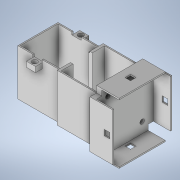
# Autodesk Inventor part: shell 2.0
Saved by Autodesk Inventor 2020.2 (Build 242310000, 310)
## iProperties
Created: 2020-02-10
Part Number: shell 2.0
Material: Generic
Document SubType Name: Modeling
Designer: ColinP
Density: 1 g/cm^3
Appearance: Default
Author: ColinP
Autodesk Inventor part; units mm, degrees
ref_plane "YZ Plane" through (0, 0, 0) normal (1, 0, 0) x (0, 1, 0)
ref_plane "XZ Plane" through (0, 0, 0) normal (0, 1, 0) x (-1, 0, 0)
ref_plane "XY Plane" through (0, 0, 0) normal (0, 0, 1) x (1, 0, 0)
sketch "Sketch1" plane through (0, 0, 0) normal (0, 1, 0) x (-1, 0, 0)
  line L0 (9.0944, 11.3049) -> (-22.9063, 11.3049)
  line L1 (9.0944, 11.3049) -> (41.0951, 11.3049) construction
  line L2 (-22.9063, 11.3049) -> (-22.9063, -19.1751)
  line L3 (-22.9063, -19.1751) -> (9.0944, -19.1751)
  line L4 (9.0944, -19.1751) -> (9.0944, 11.3049)
  point P0 (0, 0)
  dimension "d0" = 32.0007
  dimension "d1" = 180
  dimension "d2" = 30.48
  constraints: 10 end point, 2 horizontal, 2 perpendicular, 1 collinear, 1 vertical
  measures "d0" distance of L0.start L0.end
  measures "d1" angle of L0 L1
  measures "d2" distance of L0.end L2.end
extrude "Extrusion1" add sketch "Sketch1" along normal blind 2
sketch "Sketch2" plane through (0, 2, 0) normal (0, 1, 0) x (1, 0, 0)
  line L0 (-9.0944, 19.1751) -> (-9.0944, -11.3049) projected
  line L1 (-9.0944, -11.3049) -> (-9.0944, -10.3049)
  line L2 (-9.0944, -10.3049) -> (-8.0944, -10.3049)
  line L3 (-9.0944, 19.1751) -> (-8.0944, 19.1751)
  line L4 (22.9063, 19.1751) -> (-9.0944, 19.1751) projected
  line L5 (-8.0944, 19.1751) -> (-8.0944, 18.1751)
  line L6 (22.9063, 19.1751) -> (21.9063, 19.1751)
  line L7 (21.9063, 19.1751) -> (21.9063, 18.1751)
  line L8 (22.9063, -11.3049) -> (22.9063, 19.1751) projected
  line L9 (22.9063, -11.3049) -> (22.9063, -10.3049)
  line L10 (21.9063, -10.3049) -> (22.9063, -10.3049)
  line L11 (-8.0944, -10.3049) -> (21.9063, -10.3049)
  line L12 (21.9063, -10.3049) -> (21.9063, 18.1751)
  line L13 (21.9063, 18.1751) -> (-8.0944, 18.1751)
  line L14 (-8.0944, 18.1751) -> (-8.0944, -10.3049)
  line L15 (-9.0944, -11.3049) -> (22.9063, -11.3049) projected
  line L16 (22.9063, -11.3049) -> (22.9063, 19.1751) projected
  line L17 (22.9063, 19.1751) -> (-9.0944, 19.1751) projected
  line L18 (-9.0944, 19.1751) -> (-9.0944, -11.3049) projected
  line L19 (22.9063, -11.3049) -> (22.9063, -3.3649)
  line L20 (22.9063, 19.1751) -> (22.9063, 11.2351)
  line L21 (22.9063, -3.3649) -> (21.9063, -3.3649)
  line L22 (22.9063, 11.2351) -> (21.9063, 11.2351)
  point P0 (0, 0)
  point P1 (22.9063, -3.3649)
  point P2 (22.9063, 11.2351)
  dimension "d5" = 1
  dimension "d6" = 1
  dimension "d7" = 1
  dimension "d8" = 1
  dimension "d11" = 7.94
  dimension "d12" = 7.94
  constraints: 32 end point, 8 point on line, 6 perpendicular, 2 parallel, 1 horizontal, 1 vertical
  measures "d5" distance of L0.end L1.end
  measures "d6" distance of L1.end L2.end
  measures "d7" distance of L3.end L5.end
  measures "d8" distance of L4.start L6.end
  measures "d11" distance of L15.end L19.end
  measures "d12" distance of L16.end L20.end
extrude "Extrusion3" add sketch "Sketch2" along normal blind 30 contours L3 L5 L14 L2 L0 | L2 L11 L10 L8 L15 L0 | L4 L7 L13 L5 | L4 L8 L22 L12 L7 | L12 L21 L8 L10
sketch "Sketch3" plane through (0, 2, 0) normal (0, 1, 0) x (1, 0, 0)
  line L0 (21.9063, -10.3049) -> (21.9063, -3.3649) projected
  line L1 (22.9063, 11.2351) -> (21.9063, 11.2351) projected
  line L2 (21.9063, -3.3649) -> (21.9063, 11.2351)
  line L3 (21.9063, 11.2351) -> (22.9063, 11.2351)
  line L4 (22.9063, -3.3649) -> (22.9063, 11.2351) projected
  line L5 (22.9063, 11.2351) -> (22.9063, -3.3649)
  line L6 (22.9063, -3.3649) -> (21.9063, -3.3649)
  point P0 (0, 0)
  constraints: 8 end point, 3 perpendicular, 1 vertical
extrude "Extrusion4" add sketch "Sketch3" along normal blind 2
sketch "Sketch4" plane through (0, 32, 0) normal (0, 1, 0) x (1, 0, 0)
  line L0 (22.9063, -11.3049) -> (22.9063, 19.1751) projected
  line L1 (22.9063, 3.9351) -> (5.9063, 3.9351)
  line L2 (5.9063, 3.9351) -> (5.9063, 21.4351)
  line L3 (5.9063, 21.4351) -> (5.9063, -13.5649)
  circle A0 centre (5.9063, -13.5649) radius 2
  circle A1 centre (5.9063, 21.4351) radius 2
  line L4 (22.9063, 19.1751) -> (-9.0944, 19.1751) projected
  line L5 (5.9063, 19.1751) -> (2.4063, 19.1751)
  line L6 (2.4063, 19.1751) -> (2.4063, 24.1751)
  line L7 (2.4063, 24.1751) -> (9.4063, 24.1751)
  line L8 (9.4063, 24.1751) -> (9.4063, 19.1751)
  line L9 (9.4063, -11.3049) -> (9.4063, -16.3049)
  line L10 (9.4063, -16.3049) -> (2.4063, -16.3049)
  line L11 (2.4063, -16.3049) -> (2.4063, -11.3049)
  line L12 (-9.0944, -11.3049) -> (22.9063, -11.3049) projected
  point P0 (0, 0)
  dimension "d17" = 17
  dimension "d18" = 17.5
  dimension "d19" = 35
  dimension "d20" = 4
  dimension "d21" = 4
  dimension "d22" = 3.5
  dimension "d23" = 5
  dimension "d24" = 7
  dimension "d25" = 5
  constraints: 20 end point, 10 point on line, 5 perpendicular, 2 centre point, 2 coincident, 1 horizontal, 1 midpoint
  measures "d17" distance of L1.start L1.end
  measures "d18" distance of L1.end L2.end
  measures "d19" distance of L2.end L3.end
  measures "d20" diameter of A0
  measures "d21" diameter of A1
  measures "d22" distance of L5.start L5.end
  measures "d23" distance of L5.end L6.end
  measures "d24" distance of L6.end L7.end
  measures "d25" distance of L9.start L9.end
extrude "Extrusion5" add sketch "Sketch4" against normal blind 4 contours L9 L10 L11 L12 | L4 L6 L7 L8
sketch "Sketch5" plane through (0, 32, 0) normal (0, 1, 0) x (1, 0, 0)
  line L0 (2.4063, 19.1751) -> (2.4063, 24.1751) projected
  line L1 (2.4063, 19.1751) -> (2.4063, 18.1751)
  line L2 (-8.0944, 18.1751) -> (21.9063, 18.1751) projected
  line L3 (22.9063, 19.1751) -> (9.4063, 19.1751) projected
  line L4 (9.4063, 19.1751) -> (9.4063, 18.1751)
  line L5 (-9.0944, -11.3049) -> (22.9063, -11.3049) projected
  line L6 (2.4063, -11.3049) -> (2.4063, -10.3049)
  line L7 (-8.0944, -10.3049) -> (21.9063, -10.3049) projected
  line L8 (9.4063, -10.3049) -> (9.4063, -11.3049)
  circle A0 centre (5.9063, 21.4351) radius 2 projected
  circle A1 centre (5.9063, -13.5649) radius 2 projected
  line L9 (21.9063, -10.3049) -> (-8.0944, -10.3049) projected
  line L10 (-8.0944, -10.3049) -> (-8.0944, 18.1751) projected
  line L11 (-8.0944, 18.1751) -> (21.9063, 18.1751) projected
  line L12 (21.9063, 18.1751) -> (21.9063, 11.2351) projected
  line L13 (21.9063, 11.2351) -> (22.9063, 11.2351) projected
  line L14 (22.9063, 11.2351) -> (22.9063, 19.1751) projected
  line L15 (22.9063, 19.1751) -> (9.4063, 19.1751) projected
  line L16 (9.4063, 19.1751) -> (9.4063, 24.1751) projected
  line L17 (9.4063, 24.1751) -> (2.4063, 24.1751) projected
  line L18 (2.4063, 24.1751) -> (2.4063, 19.1751) projected
  line L19 (2.4063, 19.1751) -> (-9.0944, 19.1751) projected
  line L20 (-9.0944, 19.1751) -> (-9.0944, -11.3049) projected
  line L21 (-9.0944, -11.3049) -> (2.4063, -11.3049) projected
  line L22 (2.4063, -11.3049) -> (2.4063, -16.3049) projected
  line L23 (2.4063, -16.3049) -> (9.4063, -16.3049) projected
  line L24 (9.4063, -16.3049) -> (9.4063, -11.3049) projected
  line L25 (9.4063, -11.3049) -> (22.9063, -11.3049) projected
  line L26 (22.9063, -11.3049) -> (22.9063, -3.3649) projected
  line L27 (22.9063, -3.3649) -> (21.9063, -3.3649) projected
  line L28 (21.9063, -3.3649) -> (21.9063, -10.3049) projected
  point P0 (0, 0)
  point P1 (-8.0944, 18.1751)
  point P2 (22.9063, 19.1751)
  constraints: 8 end point, 4 point on line, 3 vertical, 1 perpendicular
extrude "Extrusion6" add sketch "Sketch5" along normal blind 2 contours L1 L2 L10 L7 L6 L5 L20 L19 | L4 L3 L14 L13 L12 L2 | L8 L7 L28 L27 L26 L5
sketch "Sketch7" plane through (22.9063, 0, 11.3049) normal (1, 0, 0) x (0, 0, -1)
  line L0 (0, 0) -> (30.48, 0) projected
  line L1 (15.24, 0) -> (31.74, 0)
  line L2 (15.24, 0) -> (31.74, 0) construction
  line L3 (31.74, 0) -> (-1.26, 0)
  line L4 (-1.26, 0) -> (-1.26, 35)
  line L5 (-1.26, 35) -> (31.74, 35)
  line L6 (31.74, 35) -> (31.74, 0)
  point P0 (11.3049, 0)
  dimension "d33" = 16.5
  dimension "d34" = 0
  dimension "d35" = 33
  dimension "d36" = 35
  constraints: 12 end point, 3 perpendicular, 2 collinear, 1 horizontal, 1 midpoint, 1 point on line
  measures "d33" distance of L1.start L1.end
  measures "d34" distance between parallel lines of L1 L2
  measures "d35" distance of L1.end L3.end
  measures "d36" distance of L3.end L4.end
extrude "Extrusion8" add sketch "Sketch7" along normal blind 2
sketch "Sketch8" plane through (22.9063, 0, 11.3049) normal (1, 0, 0) x (0, 0, -1)
  line L0 (-1.26, 0) -> (31.74, 0) projected
  line L1 (15.24, 0) -> (15.24, -1)
  line L2 (15.24, -1) -> (31.74, -1)
  line L3 (31.74, -1) -> (32.74, -1)
  line L4 (32.74, -1) -> (32.74, 36)
  line L5 (32.74, 36) -> (-2.26, 36)
  line L6 (-2.26, 36) -> (-2.26, -1)
  line L7 (-2.26, -1) -> (15.24, -1)
  line L8 (-1.26, 0) -> (31.74, 0) projected
  line L9 (31.74, 0) -> (31.74, 35) projected
  line L10 (31.74, 35) -> (-1.26, 35) projected
  line L11 (-1.26, 35) -> (-1.26, 0) projected
  line L12 (31.74, 0) -> (31.74, 35) projected
  line L13 (31.74, 35) -> (32.74, 35)
  line L14 (-1.26, 35) -> (-2.26, 35)
  point P0 (11.3049, 0)
  dimension "d39" = 1
  dimension "d40" = 1
  dimension "d41" = 37
  dimension "d42" = 35
  constraints: 18 end point, 6 perpendicular, 4 point on line, 1 midpoint, 1 parallel, 1 vertical
  measures "d39" distance of L1.start L1.end
  measures "d40" distance of L2.end L3.end
  measures "d41" distance of L3.end L4.end
  measures "d42" distance of L4.end L5.end
extrude "Extrusion9" add sketch "Sketch8" along normal blind 30 contours L0 L1 L7 L6 L14 L11 | L0 L9 L13 L4 L3 L2 L1
sketch "Sketch9" plane through (52.9063, 0, 11.3049) normal (1, 0, 0) x (0, 0, -1)
  line L0 (32.74, -1) -> (32.74, 35) projected
  line L1 (-2.26, -1) -> (32.74, -1) projected
  line L2 (-2.26, 35) -> (-2.26, -1) projected
  line L3 (31.74, 35) -> (-1.26, 35) projected
  line L4 (-1.26, 35) -> (-2.26, 35) projected
  line L5 (32.74, 35) -> (31.74, 35) projected
  point P0 (11.3049, 0)
sketch "Sketch10" plane through (22.9063, 35, 13.5649) normal (0, 1, 0) x (1, 0, 0)
  line L0 (0, 2.26) -> (0, 10.2) projected
  line L1 (0, 10.2) -> (2, 10.2)
  line L2 (2, 1) -> (2, 34) projected
  line L3 (-1, 24.8) -> (0, 24.8) projected
  line L4 (0, 24.8) -> (2, 24.8)
  line L5 (2, 24.8) -> (2, 10.2)
  line L6 (0, 10.2) -> (-1, 10.2) projected
  line L7 (0, 10.2) -> (0, 24.8)
  point P0 (-22.9063, 13.5649)
  point P1 (2, 24.8)
  constraints: 8 end point, 2 horizontal, 2 perpendicular, 1 point on line
extrude "Extrusion11" cut sketch "Sketch10" against normal blind 31
sketch "Sketch14" plane through (0, 0, 0) normal (0, -1, 0) x (1, 0, 0)
  line L0 (22.9063, -19.1751) -> (22.9063, 11.3049) projected
  line L1 (-9.0944, 11.3049) -> (22.9063, 11.3049) projected
  line L2 (-9.0944, -19.1751) -> (-9.0944, 11.3049) projected
  line L3 (22.9063, -19.1751) -> (-9.0944, -19.1751) projected
  point P0 (0, 0)
extrude "Extrusion13" add sketch "Sketch14" along normal up to surface (1 mm away)
sketch "Sketch15" plane through (0, 2, 0) normal (0, 1, 0) x (1, 0, 0)
  line L0 (21.9063, -10.3049) -> (21.9063, 18.1751) projected
  line L1 (21.9063, 18.1751) -> (-8.0944, 18.1751) projected
  line L2 (-8.0944, 18.1751) -> (-8.0944, -10.3049) projected
  line L3 (-8.0944, -10.3049) -> (21.9063, -10.3049) projected
  point P0 (0, 0)
extrude "Extrusion14" cut sketch "Sketch15" against normal blind 2
extrude "Extrusion16" add sketch "Sketch9" along normal blind 2
sketch "Sketch17" plane through (52.9063, 0, 11.3049) normal (-1, 0, 0) x (0, 0, 1)
  line L0 (-31.74, 0) -> (-31.74, 3)
  line L1 (-31.74, 3) -> (-29.89, 3)
  line L2 (-29.89, 3) -> (-29.89, 32.7)
  line L3 (-29.89, 32.7) -> (-0.59, 32.7)
  line L4 (-0.59, 32.7) -> (-0.59, 3)
  line L5 (-29.89, 32.7) -> (-28.24, 32.7)
  line L6 (-0.59, 32.7) -> (-2.19, 32.7)
  line L7 (-0.59, 3) -> (-2.19, 3)
  line L8 (-29.89, 3) -> (-28.24, 3)
  point P0 (-11.3049, 0)
  dimension "d69" = 3
  dimension "d70" = 1.85
  dimension "d71" = 29.7
  dimension "d72" = 29.3
  dimension "d73" = 29.7
  dimension "d74" = 90
  dimension "d112" = 1.65
  dimension "d113" = 1.6
  dimension "d114" = 1.6
  dimension "d115" = 1.65
  constraints: 18 end point, 4 perpendicular, 2 horizontal, 2 point on line, 1 vertical
  measures "d69" distance of L0.start L0.end
  measures "d70" distance of L0.end L1.end
  measures "d71" distance of L1.end L2.end
  measures "d72" distance of L2.end L3.end
  measures "d73" distance of L3.end L4.end
  measures "d74" angle of L3 L4
  measures "d112" distance of L2.end L5.end
  measures "d113" distance of L3.end L6.end
  measures "d114" distance of L4.end L7.end
  measures "d115" distance of L1.end L8.end
sketch "Sketch18" plane through (54.9063, 0, 11.3049) normal (1, 0, 0) x (0, 0, -1)
  line L0 (32.74, 35) -> (-2.26, 35) projected
  line L1 (-2.26, 35) -> (-2.26, -1) projected
  line L2 (-2.26, -1) -> (32.74, -1) projected
  line L3 (32.74, -1) -> (32.74, 35) projected
  line L4 (32.74, 35) -> (37.74, 35)
  line L5 (37.74, 35) -> (37.74, -1)
  line L6 (37.74, -1) -> (32.74, -1)
  line L7 (-2.26, -1) -> (0, -1) projected
  line L8 (-2.26, -1) -> (-7.26, -1)
  line L9 (-7.26, -1) -> (-7.26, 35)
  line L10 (-7.26, 35) -> (-2.26, 35)
  line L11 (37.74, 35) -> (36.74, 35)
  line L12 (36.74, 35) -> (36.74, -1)
  line L13 (-7.26, -1) -> (-6.26, -1)
  line L14 (-6.26, -1) -> (-6.26, 35)
  line L15 (36.74, -1) -> (36.74, 0)
  line L16 (36.74, 0) -> (32.74, 0)
  line L17 (32.74, -1) -> (32.74, 35) projected
  line L18 (-2.26, 35) -> (-2.26, -1) projected
  line L19 (-2.26, 0) -> (-6.26, 0)
  line L20 (-6.26, 35) -> (-6.26, 34)
  line L21 (-6.26, 34) -> (-2.26, 34)
  line L22 (32.74, 34) -> (36.74, 34)
  point P0 (11.3049, 0)
  dimension "d75" = 5
  dimension "d76" = 5
  dimension "d77" = 1
  dimension "d78" = 1
  dimension "d79" = 1
  dimension "d80" = 1
  constraints: 32 end point, 17 point on line, 6 perpendicular, 1 collinear, 1 horizontal, 1 vertical
  measures "d75" distance of L0.start L4.end
  measures "d76" distance of L1.end L8.end
  measures "d77" distance of L4.end L11.end
  measures "d78" distance of L8.end L13.end
  measures "d79" distance of L12.end L15.end
  measures "d80" distance of L14.end L20.end
extrude "Extrusion17" add sketch "Sketch18" along normal blind 2 contours L4 L12 L22 L3 | L1 L21 L14 L10 | L22 L12 L16 L3 | L1 L19 L14 L21 | L16 L12 L6 L3 | L1 L8 L14 L19
extrude "Extrusion18" add sketch "Sketch18" along normal blind 15 contours L4 L5 L6 L12 | L14 L8 L9 L10
sketch "Sketch19" plane through (54.9063, 0, 11.3049) normal (-1, 0, 0) x (0, 0, 1)
  line L0 (7.26, -1) -> (2.26, -1) projected
  line L1 (7.26, 35) -> (7.26, -1) projected
  line L2 (2.26, 35) -> (7.26, 35) projected
  line L3 (2.26, 35) -> (2.26, -1) projected
  line L4 (-32.74, -1) -> (-37.74, -1) projected
  line L5 (-32.74, -1) -> (-32.74, 35) projected
  line L6 (-37.74, 35) -> (-32.74, 35) projected
  line L7 (-37.74, -1) -> (-37.74, 35) projected
  point P0 (-11.3049, 0)
extrude "Extrusion19" add sketch "Sketch19" along normal blind 2
sketch "Sketch20" plane through (54.9063, 0, 11.3049) normal (1, 0, 0) x (0, 0, -1)
  line L0 (-2.26, -1) -> (-2.26, 35) projected
  line L1 (-2.26, -1) -> (-2.26, -6)
  line L2 (-2.26, -6) -> (32.74, -6)
  line L3 (32.74, 35) -> (32.74, -1) projected
  line L4 (32.74, -6) -> (32.74, -1)
  line L5 (32.74, -1) -> (32.74, -5)
  line L6 (32.74, -5) -> (-2.26, -5)
  line L7 (-2.26, -1) -> (32.74, -1) projected
  line L8 (36.74, 35) -> (32.74, 35) projected
  line L9 (32.74, -1) -> (32.74, 35)
  line L10 (32.74, 35) -> (32.74, 40)
  line L11 (32.74, 40) -> (-2.26, 40)
  line L12 (-2.26, 40) -> (-2.26, 35)
  line L13 (-2.26, 35) -> (-2.26, 40)
  line L14 (-2.26, 40) -> (-2.26, 39)
  line L15 (-2.26, 39) -> (32.74, 39)
  point P0 (11.3049, 0)
  dimension "d87" = 5
  dimension "d88" = 4
  dimension "d89" = 5
  dimension "d90" = 1
  constraints: 24 end point, 7 perpendicular, 7 point on line, 1 collinear, 1 vertical
  measures "d87" distance of L0.start L1.end
  measures "d88" distance of L3.end L5.end
  measures "d89" distance of L3.start L10.end
  measures "d90" distance of L11.end L14.end
extrude "Extrusion20" add sketch "Sketch20" along normal blind 15 contours L6 L4 L2 L1 | L12 L11 L10 L15
extrude "Extrusion21" add sketch "Sketch20" against normal blind 2 contours L7 L4 L6 L1 | L0 L12 L15 L10 L3 L7
sketch "Sketch21" plane through (69.9063, -1, 18.5649) normal (0, 0, 1) x (1, 0, 0)
  line L0 (0, 36) -> (0, 0) projected
  line L1 (0, 0) -> (0, 18)
  line L2 (0, 18) -> (-2, 18)
  line L3 (-2, 18) -> (-6.2, 18)
  line L4 (-6.2, 18) -> (-6.2, 20.1)
  line L5 (-6.2, 20.1) -> (-2, 20.1)
  line L6 (-2, 20.1) -> (-2, 15.9)
  line L7 (-2, 15.9) -> (-6.2, 15.9)
  line L8 (-6.2, 15.9) -> (-6.2, 18)
  point P0 (-69.9063, 1)
  dimension "d95" = 18
  dimension "d96" = 2
  dimension "d97" = 4.2
  dimension "d98" = 2.1
  dimension "d99" = 4.2
  constraints: 16 end point, 6 perpendicular, 2 point on line, 1 midpoint
  measures "d95" distance of L0.end L1.end
  measures "d96" distance of L1.end L2.end
  measures "d97" distance of L2.end L3.end
  measures "d98" distance of L3.end L4.end
  measures "d99" distance of L5.end L6.end
extrude "Extrusion22" cut sketch "Sketch21" against normal through all
sketch "Sketch22" plane through (54.9063, 40, 13.5649) normal (0, 1, 0) x (1, 0, 0)
  line L0 (15, 0) -> (15, 35) projected
  line L1 (15, 0) -> (15, 18)
  line L2 (15, 18) -> (13, 18)
  line L3 (13, 18) -> (8.8, 18)
  line L4 (8.8, 18) -> (7.8, 18)
  line L5 (7.8, 18) -> (3.6, 18)
  line L6 (7.8, 18) -> (7.8, 20.1)
  line L7 (7.8, 20.1) -> (3.6, 20.1)
  line L8 (3.6, 20.1) -> (3.6, 15.9)
  line L9 (3.6, 15.9) -> (7.8, 15.9)
  line L10 (7.8, 15.9) -> (7.8, 18)
  point P0 (-54.9063, 13.5649)
  dimension "d102" = 18
  dimension "d103" = 2
  dimension "d104" = 4.2
  dimension "d105" = 1
  dimension "d106" = 4.2
  dimension "d107" = 2.1
  dimension "d108" = 4.2
  dimension "d109" = 4.2
  constraints: 20 end point, 5 perpendicular, 5 point on line, 1 vertical
  measures "d102" distance of L0.start L1.end
  measures "d103" distance of L1.end L2.end
  measures "d104" distance of L2.end L3.end
  measures "d105" distance of L3.end L4.end
  measures "d106" distance of L4.end L5.end
  measures "d107" distance of L4.end L6.end
  measures "d108" distance of L6.end L7.end
  measures "d109" distance of L7.end L8.end
extrude "Extrusion23" cut sketch "Sketch22" against normal through all
hole "Hole1" at (52.9063, 32.7, 9.1149) at (52.9063, 3, 9.1149) at (52.9063, 3, -16.9351) at (52.9063, 32.7, -16.9351) direction (1, 0, 0) diameter 3.4 end through all
sketch "Sketch23" plane through (54.9063, 0, 11.3049) normal (-1, 0, 0) x (0, 0, 1)
  line L0 (-32.74, -5) -> (2.26, -5) projected
  line L1 (-32.74, -6) -> (-32.74, -5) projected
  line L2 (2.26, -6) -> (-32.74, -6) projected
  line L3 (2.26, -5) -> (2.26, -6) projected
  line L4 (-32.74, 39) -> (-32.74, 40) projected
  line L5 (2.26, 39) -> (-32.74, 39) projected
  line L6 (2.26, 40) -> (2.26, 39) projected
  line L7 (-32.74, 40) -> (2.26, 40) projected
  point P0 (-11.3049, 0)
extrude "Extrusion24" add sketch "Sketch23" along normal blind 2
sketch "Sketch24" plane through (54.9063, 0, 11.3049) normal (1, 0, 0) x (0, 0, -1)
  circle A0 centre (28.24, 3) radius 1.7 projected
  circle A1 centre (2.19, 32.7) radius 1.7 projected
  circle A2 centre (2.19, 3) radius 1.7 projected
  circle A3 centre (28.24, 32.7) radius 1.7 projected
  line L0 (-2.26, 35) -> (-2.26, -1) projected
  line L1 (-2.26, -1) -> (-2.26, -5) projected
  line L2 (32.74, -5) -> (-2.26, -5) projected
  line L3 (32.74, -5) -> (32.74, -1) projected
  line L4 (32.74, -1) -> (32.74, 35) projected
  line L5 (32.74, 35) -> (32.74, 39) projected
  line L6 (-2.26, 39) -> (32.74, 39) projected
  line L7 (-2.26, 39) -> (-2.26, 35) projected
  point P0 (11.3049, 0)
extrude "Extrusion25" add sketch "Sketch24" along normal blind 2
body "Solid1"
